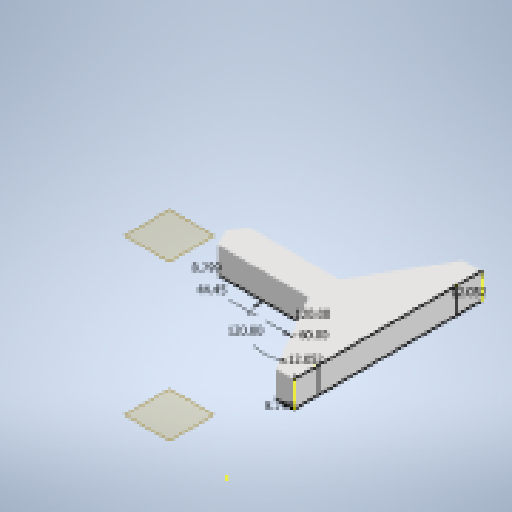
# Autodesk Inventor part: HorizontalGrabberMain
Saved by Autodesk Inventor 2024.2 (Build 282272000, 272)
## iProperties
Created: 2024-02-28
Part Number: HorizontalGrabberMain
Material: Generic
Document SubType Name: Modeling
Designer: Jared
Density: 1 g/cm^3
Appearance: Default
Author: Jared
Autodesk Inventor part; units mm, degrees
ref_plane "YZ Plane" through (0, 0, 0) normal (1, 0, 0) x (0, 1, 0)
ref_plane "XZ Plane" through (0, 0, 0) normal (0, 1, 0) x (-1, 0, 0)
ref_plane "XY Plane" through (0, 0, 0) normal (0, 0, 1) x (1, 0, 0)
ref_plane "Work Plane1" through (0, 12.7, 0) normal (0, 1, 0) x (1, 0, 0)
sketch "Sketch3" plane through (0, 12.7, 0) normal (0, 1, 0) x (1, 0, 0)
  line L0 (19.05, 32.9956) -> (-3.175, 71.4904)
  line L1 (19.05, 32.9956) -> (27.8488, 32.9956)
  line L2 (-47.625, 71.4904) -> (-52.0244, 79.1104)
  line L3 (27.8488, 32.9956) -> (27.8488, 32.9956)
  line L4 (27.8488, 32.9956) -> (27.8488, 32.9956)
  line L5 (1.2244, 79.1104) -> (-3.175, 71.4904)
  line L6 (-3.175, 71.4904) -> (-47.625, 71.4904)
  line L7 (1.2244, 79.1104) -> (27.8488, 32.9956)
  line L8 (27.8488, 32.9956) -> (19.05, 32.9956)
  line L9 (27.8488, 32.9956) -> (27.8488, 32.9956)
  line L10 (27.8488, 32.9956) -> (27.8488, 32.9956)
  line L11 (1.2244, 79.1104) -> (-52.0244, 79.1104)
  line L12 (19.05, 125.2252) -> (-3.175, 86.7304)
  line L13 (19.05, 125.2252) -> (27.8488, 125.2252)
  line L14 (-47.625, 86.7304) -> (-52.0244, 79.1104)
  line L15 (27.8488, 125.2252) -> (27.8488, 125.2252)
  line L16 (27.8488, 125.2252) -> (27.8488, 125.2252)
  line L17 (1.2244, 79.1104) -> (-3.175, 86.7304)
  line L18 (-3.175, 86.7304) -> (-47.625, 86.7304)
  line L19 (1.2244, 79.1104) -> (27.8488, 125.2252)
  line L20 (27.8488, 125.2252) -> (19.05, 125.2252)
  line L21 (27.8488, 125.2252) -> (27.8488, 125.2252)
  line L22 (27.8488, 125.2252) -> (27.8488, 125.2252)
  line L23 (27.8488, 32.9956) -> (27.8488, 125.2252)
  point P0 (-38.1, 71.4904)
  dimension "d53" = 8.7988
  dimension "d54" = 8.7988
  dimension "d59" = 90
  dimension "d60" = 120
  dimension "d62" = 120
  dimension "d163" = 44.45
  dimension "d173" = 60
  constraints: 48 end point, 9 symmetric about line, 8 point on line, 4 horizontal, 3 equal length, 1 parallel, 1 perpendicular, 1 vertical, 1 other
  measures "d53" distance of L0.start L1.end
  measures "d54" distance of L2.start L2.end
  measures "d59" angle of L4 L3
  measures "d60" angle of L6 L0
  measures "d62" angle of L5 L6
  measures "d163" distance of L0.end L2.start
  measures "d173" angle of L7 L5
ref_plane "Work Plane2" through (0, 88.9, 0) normal (0, 1, 0) x (1, 0, 0)
extrude "Extrusion11" add sketch "Sketch3" along normal blind 12.7 contours L0 L5 L7 L1 | L6 L2 L11 L5
extrude "Extrusion21" add sketch "Sketch3" along normal blind 12.7 contours L11 L14 L18 L17 | L17 L12 L13 L19
extrude "Extrusion22" add sketch "Sketch3" along normal blind 12.7 contours L7 L19 L23
sketch "Sketch15" plane through (27.8488, 12.7, -32.9956) normal (1, 0, 0) x (0, 0, -1)
  line L0 (0, 0) -> (0, 12.7) projected
  line L1 (0, 12.7) -> (12.0516, 12.7)
  line L2 (0, 12.7) -> (92.2297, 12.7) projected
  line L3 (92.2297, 0) -> (92.2297, 12.7) projected
  line L4 (92.2297, 12.7) -> (80.1781, 12.7)
  line L5 (12.0516, 12.7) -> (12.0516, 0)
  line L6 (38.4948, 0) -> (0, 0) projected
  line L7 (80.1781, 12.7) -> (80.1781, 0)
  line L8 (80.1781, 0) -> (12.0516, 0)
  line L9 (12.0516, 12.7) -> (80.1781, 12.7)
  point P0 (-32.9956, -12.7)
  point P1 (38.4948, 0)
  dimension "d180" = 12.0516
  dimension "d181" = 12.0516
  constraints: 12 end point, 3 point on line, 2 collinear, 2 vertical
  measures "d180" distance of L0.end L1.end
  measures "d181" distance of L2.end L4.end
extrude "Extrusion23" add sketch "Sketch15" along normal blind 22.86 contours L5 L2 L7 L8 L6
sketch "Sketch16" plane through (0, 25.4, 0) normal (0, 1, 0) x (1, 0, 0)
  line L0 (27.8488, 45.0472) -> (50.7088, 45.0472) projected
  line L1 (50.7088, 45.0472) -> (50.7088, 55.0472)
  line L2 (50.7088, 113.1736) -> (50.7088, 45.0472) projected
  line L3 (27.8488, 32.9956) -> (27.8488, 45.0472) projected
  line L4 (27.8488, 45.0472) -> (27.8488, 55.0472)
  line L5 (27.8488, 55.0472) -> (50.7088, 55.0472)
  line L6 (27.8488, 45.0472) -> (17.8488, 45.0472)
  line L7 (17.8488, 45.0472) -> (17.8488, 55.0472)
  line L8 (17.8488, 55.0472) -> (27.8488, 55.0472)
  point P0 (0, 0)
  dimension "d184" = 10
  dimension "d185" = 10
  dimension "d199" = 10
  dimension "d200" = 10
  constraints: 12 end point, 1 horizontal, 1 perpendicular, 1 point on line, 1 vertical
  measures "d184" distance of L0.end L1.end
  measures "d185" distance of L0.start L4.end
  measures "d199" distance of L0.start L6.end
  measures "d200" distance of L6.end L7.end
extrude "Extrusion24" add sketch "Sketch16" along normal blind 18.288
sketch "Sketch18" plane through (27.8488, 12.7, -45.0472) normal (0, 0, 1) x (1, 0, 0)
  line L0 (-7, 22.988) -> (-7, 30.988) projected
  line L1 (-7, 30.988) -> (-7, 22.988)
  line L2 (-7, 22.988) -> (3.1943, 22.988)
  line L3 (3.1943, 22.988) -> (3.1943, 30.988)
  line L4 (3.1943, 30.988) -> (-7, 30.988)
  point P0 (-27.8488, -12.7)
  constraints: 8 end point, 3 perpendicular, 1 collinear
extrude "Extrusion26" add sketch "Sketch18" along normal blind 48
sketch "Sketch19" plane through (50.7088, 12.7, -32.9956) normal (1, 0, 0) x (0, 0, -1)
  line L0 (12.0516, 30.988) -> (22.0516, 30.988) projected
  line L1 (12.0516, 22.988) -> (22.0516, 22.988) projected
  line L2 (12.0516, 30.988) -> (12.0516, 22.988)
  line L3 (12.0516, 22.988) -> (22.0516, 22.988)
  line L4 (22.0516, 22.988) -> (22.0516, 30.988)
  line L5 (22.0516, 30.988) -> (12.0516, 30.988)
  point P0 (-32.9956, -12.7)
  constraints: 8 end point, 2 perpendicular, 1 collinear, 1 vertical
extrude "Extrusion27" add sketch "Sketch19" along normal blind 8
sketch "Sketch20" plane through (27.8488, 12.7, -45.0472) normal (0, 0, 1) x (1, 0, 0)
  line L0 (-10, 30.988) -> (30.86, 30.988) projected
  line L1 (30.86, 30.988) -> (23.2839, 30.988)
  line L2 (30.86, 30.988) -> (30.86, 22.988) projected
  line L3 (30.86, 30.988) -> (30.86, 22.988)
  line L4 (23.2839, 30.988) -> (23.2839, 22.988)
  line L5 (22.86, 22.988) -> (30.86, 22.988) projected
  line L6 (23.2839, 22.988) -> (30.86, 22.988)
  point P0 (-27.8488, -12.7)
  point P1 (-7, 30.988)
  constraints: 8 end point, 1 collinear, 1 perpendicular, 1 point on line, 1 vertical
extrude "Extrusion28" add sketch "Sketch20" along normal blind 48
sketch "Sketch21" plane through (31.0431, 35.688, -45.0472) normal (1, 0, 0) x (0, 0, -1)
  line L0 (0, 8) -> (-48, 8) projected
  line L1 (-48, 8) -> (-40.0559, 8)
  line L2 (0, 0) -> (-48, 0) projected
  line L3 (-48, 8) -> (-40.0559, 8)
  line L4 (-40.0559, 8) -> (-40.0559, 0)
  line L5 (-40.0559, 0) -> (-48, 0)
  line L6 (-48, 0) -> (-48, 8)
  point P0 (-45.0472, -35.688)
  point P1 (-40.0559, 8)
  constraints: 10 end point, 2 parallel, 2 point on line, 1 horizontal, 1 perpendicular
extrude "Extrusion29" add sketch "Sketch21" along normal blind 24
sketch "Sketch22" plane through (20.8488, 35.688, -45.0472) normal (0, -1, 0) x (1, 0, 0)
  line L0 (29.86, -10) -> (29.86, 0) projected
  line L1 (29.86, 0) -> (29.86, -10)
  line L2 (-3, -10) -> (37.86, -10) projected
  line L3 (29.86, -10) -> (37.86, -10)
  line L4 (37.86, -10) -> (37.86, 0)
  line L5 (37.86, -10) -> (37.86, 48) projected
  line L6 (37.86, 0) -> (29.86, 0)
  line L7 (10.1943, 0) -> (30.2839, 0) projected
  point P0 (-20.8488, 45.0472)
  constraints: 8 end point, 2 collinear, 1 perpendicular, 1 point on line
extrude "Extrusion30" add sketch "Sketch22" along normal blind 0.1
sketch "Sketch23" plane through (27.8488, 12.7, -125.2252) normal (1, 0, 0) x (0, 0, -1)
  line L0 (0, 12.7) -> (-38.4948, 12.7) projected
  line L1 (0, 12.7) -> (-92.23, 12.7)
  line L2 (-92.23, 12.7) -> (-46.115, 12.7)
  line L3 (-46.115, 12.7) -> (-46.115, -5.4256)
  point P0 (-125.2252, -12.7)
  dimension "d206" = 92.23
  dimension "d207" = 46.115
  constraints: 6 end point, 1 collinear, 1 midpoint, 1 perpendicular
  measures "d206" distance of L0.start L1.end
  measures "d207" distance of L1.end L2.end
ref_plane "Work Plane5" through (27.8488, 25.4, -79.1102) normal (0, 0, 1) x (0, -1, 0)
mirror "Mirror2" about plane through (27.8488, 25.4, -79.1102) normal (0, 0, 1) of "Extrusion24", "Extrusion26", "Extrusion27", "Extrusion28", "Extrusion29", "Extrusion30"
sketch "Sketch24" plane through (0, 25.4, 0) normal (0, 1, 0) x (1, 0, 0)
  line L0 (50.7088, 103.1733) -> (50.7088, 55.0472) projected
  line L1 (50.7088, 55.0472) -> (50.7088, 103.1733)
  line L2 (50.7088, 103.1733) -> (40.7088, 103.1733)
  line L3 (58.7088, 103.1733) -> (17.8488, 103.1733) projected
  line L4 (40.7088, 103.1733) -> (40.7088, 55.0472)
  line L5 (17.8488, 55.0472) -> (50.7088, 55.0472) projected
  line L6 (40.7088, 55.0472) -> (50.7088, 55.0472)
  point P0 (0, 0)
  dimension "d209" = 10
  dimension "d210" = 90
  constraints: 8 end point, 2 point on line, 1 collinear, 1 vertical
  measures "d209" distance of L0.start L2.end
  measures "d210" angle of L4 L2
extrude "Extrusion31" add sketch "Sketch24" along normal blind 24
sketch "Sketch25" plane through (40.7088, 25.4, -103.1733) normal (-1, 0, 0) x (0, 0, 1)
  line L0 (0, 18.288) -> (0, 24) projected
  line L1 (48.1261, 0) -> (0, 0) projected
  line L2 (0, 24) -> (48.1261, 24)
  line L3 (48.1261, 24) -> (48.1261, 0)
  line L4 (48.1261, 0) -> (0, 0)
  line L5 (0, 0) -> (0, 24)
  line L6 (0, 24) -> (24.0631, 24)
  line L7 (24.0631, 24) -> (24.0631, 12)
  circle A0 centre (24.0631, 12) radius 1.55
  line L8 (24.0631, 12) -> (24.0631, 20)
  circle A1 centre (24.0631, 20) radius 1.55
  line L9 (24.0631, 12) -> (24.0631, 4)
  circle A2 centre (24.0631, 4) radius 1.55
  line L10 (24.0631, 12) -> (16.0631, 12)
  line L11 (16.0631, 12) -> (32.0631, 12)
  circle A3 centre (16.0631, 12) radius 1.55
  circle A4 centre (32.0631, 12) radius 1.55
  circle A5 centre (0.0631, 12) radius 1.55
  circle A6 centre (8.0631, 12) radius 1.55
  circle A7 centre (8.0631, 20) radius 1.55
  circle A8 centre (16.0631, 12) radius 1.55
  circle A9 centre (8.0631, 4) radius 1.55
  circle A10 centre (32.0631, 12) radius 1.55
  circle A11 centre (40.0631, 12) radius 1.55
  circle A12 centre (40.0631, 20) radius 1.55
  circle A13 centre (48.0631, 12) radius 1.55
  circle A14 centre (40.0631, 4) radius 1.55
  circle A15 centre (16.0631, 12) radius 1.55
  circle A16 centre (24.0631, 12) radius 1.55
  circle A17 centre (24.0631, 20) radius 1.55
  circle A18 centre (32.0631, 12) radius 1.55
  circle A19 centre (24.0631, 4) radius 1.55
  point P0 (103.1733, -25.4)
  dimension "d216" = 3.1
  dimension "d217" = 8
  dimension "d218" = 3.1
  dimension "d219" = 8
  dimension "d220" = 3.1
  dimension "d221" = 8
  dimension "d222" = 16
  dimension "d223" = 3.1
  dimension "d224" = 3.1
  dimension "d229" = 16
  dimension "d232" = 16
  constraints: 20 centre point, 20 end point, 5 coincident, 4 horizontal, 2 parallel, 2 point on line, 2 vertical, 1 midpoint, 1 perpendicular, 30 other
  measures "d216" diameter of A0
  measures "d217" distance of L8.start L8.end
  measures "d218" diameter of A1
  measures "d219" distance of L8.start L9.end
  measures "d220" diameter of A2
  measures "d221" distance of L8.start L10.end
  measures "d222" distance of L10.end L11.end
  measures "d223" diameter of A3
  measures "d224" diameter of A4
  measures "d229" distance of A3.centre A5.centre
  measures "d232" distance of A3.centre A10.centre
extrude "Extrusion32" cut sketch "Sketch25" against normal blind 14.75 contours A4 | A2 | A3 | A0 L11 L7 | L7 L10 A0 | A1 L7 | L7 A1 | L11 A0 L9 | L9 A0 L10 | A6 | A7 | A9 | A11 | A12 | A14
body "Solid5"
